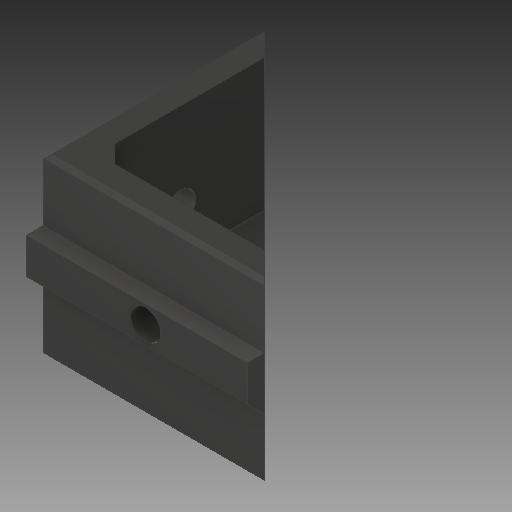
# Autodesk Inventor part: Corner Bracket
Saved by Autodesk Inventor 2019 (Build 230136000, 136)
## iProperties
Created: 2018-10-13
Part Number: Corner Bracket
Material: ABS Plastic
Document SubType Name: Modeling
Designer: Ax
Density: 1.06 g/cm^3
Appearance: Smooth - Black
Mass: 3.65093 g
Surface Area: 25.2526 cm^2
Volume: 3.44427 cm^3
Author: Ax
Autodesk Inventor part; units mm, degrees
ref_plane "YZ Plane" through (0, 0, 0) normal (1, 0, 0) x (0, 1, 0)
ref_plane "XZ Plane" through (0, 0, 0) normal (0, 1, 0) x (-1, 0, 0)
ref_plane "XY Plane" through (0, 0, 0) normal (0, 0, 1) x (1, 0, 0)
sketch "Sketch1" plane through (0, 0, 0) normal (0, 1, 0) x (-1, 0, 0)
  line L0 (-12.5, 12.5) -> (12.5, 12.5)
  line L1 (12.5, 12.5) -> (12.5, -12.5)
  line L2 (12.5, -12.5) -> (-12.5, -12.5)
  line L3 (-12.5, -12.5) -> (-12.5, 12.5)
  line L4 (-12.5, 12.5) -> (12.5, -12.5)
  line L5 (12.5, 12.5) -> (-12.5, -12.5) construction
  point P0 (0, 0)
  point P1 (0, 0)
  point P2 (0, 0)
  dimension "d0" = 25
  constraints: 12 end point, 3 midpoint, 2 parallel, 2 perpendicular, 1 coincident, 1 horizontal
  measures "d0" distance of L1.end L2.end
extrude "Extrusion1" add sketch "Sketch1" along normal blind 20 contours L0 L1 L4
sketch "Sketch2" plane through (0, 20, 0) normal (0, 1, 0) x (1, 0, 0)
  line L0 (9.5, 9.5) -> (-9.5, 9.5)
  line L1 (-9.5, 9.5) -> (-9.5, -9.5)
  line L2 (-9.5, -9.5) -> (9.5, -9.5)
  line L3 (9.5, -9.5) -> (9.5, 9.5)
  line L4 (9.5, 9.5) -> (-9.5, -9.5) construction
  line L5 (-9.5, 9.5) -> (9.5, -9.5) construction
  line L6 (-12.5, 12.5) -> (-12.5, -12.5) projected
  line L7 (-12.5, -12.5) -> (12.5, -12.5) projected
  point P0 (0, 0)
  dimension "d3" = 3
  dimension "d4" = 3
  constraints: 12 end point, 2 midpoint, 2 parallel, 1 horizontal, 1 perpendicular
  measures "d3" distance between parallel lines of L6 L1
  measures "d4" distance between parallel lines of L7 L2
extrude "Extrusion2" cut sketch "Sketch2" against normal blind 17
sketch "Sketch5" plane through (-12.5, 0, 12.5) normal (0, 0, 1) x (1, 0, 0)
  line L0 (0, 0) -> (0, 20) construction
  line L1 (0, 10) -> (25, 10) construction
  line L2 (25, 8) -> (0, 8)
  line L3 (0, 8) -> (0, 12)
  line L4 (0, 12) -> (25, 12)
  line L5 (25, 12) -> (25, 8)
  line L6 (25, 8) -> (0, 12) construction
  line L7 (0, 8) -> (25, 12) construction
  line L8 (25, 0) -> (25, 20) projected
  point P0 (12.5, 0)
  point P1 (12.5, 10)
  dimension "d22" = 4
  constraints: 14 end point, 4 midpoint, 2 horizontal, 2 parallel, 2 point on line, 1 perpendicular
  measures "d22" distance of L3.end L2.end
extrude "Extrusion5" add sketch "Sketch5" along normal blind 1
sketch "Sketch6" plane through (-12.5, 0, -12.5) normal (-1, 0, 0) x (0, 0, 1)
  line L0 (25, 8) -> (26, 8) projected
  line L1 (26, 8) -> (0, 8)
  line L2 (0, 8) -> (0, 12)
  line L3 (0, 12) -> (26, 12)
  line L4 (26, 12) -> (26, 8)
  line L5 (0, 0) -> (0, 20) projected
  point P0 (12.5, 0)
  constraints: 8 end point, 2 parallel, 1 coincident, 1 horizontal, 1 perpendicular, 1 point on line
extrude "Extrusion6" add sketch "Sketch6" along normal blind 1
chamfer "Chamfer4" distance 1 angle 45 4 edges at (-12.5, 12, 0) (0, 12, 12.5) (0, 8, 12.5) (-12.5, 8, 0)
sketch "Sketch7" plane through (9.5, 20, 9.5) normal (0, 0, -1) x (-1, 0, 0)
  line L0 (19, 0) -> (19, -17) construction
  line L1 (23, -12) -> (23, -8) projected
  line L2 (23, -10) -> (-3, -10) construction
  line L3 (9.5, -20) -> (9.5, 0) construction
  line L4 (0, 0) -> (19, 0) projected
  circle A0 centre (9.5, -10) radius 1.7
  dimension "d30" = 3.4
  constraints: 6 end point, 3 midpoint, 1 centre point, 1 horizontal
  measures "d30" diameter of A0
extrude "Extrusion7" cut sketch "Sketch7" against normal through all
sketch "Sketch8" plane through (-9.5, 20, 9.5) normal (1, 0, 0) x (0, 0, -1)
  line L0 (9.5, -20) -> (9.5, 0) construction
  line L1 (0, 0) -> (19, 0) projected
  line L2 (-1.6609, -10) -> (22, -10) construction
  line L3 (22, -13) -> (22, -7) projected
  circle A0 centre (9.5, -10) radius 1.7
  dimension "d33" = 3.4
  constraints: 4 end point, 3 midpoint, 1 centre point, 1 horizontal, 1 point on line
  measures "d33" diameter of A0
extrude "Extrusion8" cut sketch "Sketch8" against normal through all
chamfer "Chamfer5" distance 1 angle 45 2 edges at (12.5, 10, 13.5) (-13.5, 10, -12.5)
chamfer "Chamfer6" distance 2 angle 45 3 edges at (-9.5, 11.5, 9.5) (-9.5, 3, 0) (0, 3, 9.5)
chamfer "Chamfer7" distance 0.5 angle 45 5 edges at (-12.5, 0, 0) (0, 0, 12.5) (0, 0, 0) (-12.5, 20, 0) (0, 20, 12.5)
body "Solid1"
